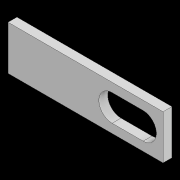
# Autodesk Inventor part: Platina Posterior Derecha
Saved by Autodesk Inventor 2021 (Build 250183000, 183)
## iProperties
Created: 2021-04-25
Part Number: Platina Posterior Derecha
Material: Generic
Document SubType Name: Modeling
Designer: maaro
Density: 1 g/cm^3
Appearance: Default
Author: maaro
Autodesk Inventor part; units mm, degrees
ref_plane "YZ Plane" through (0, 0, 0) normal (1, 0, 0) x (0, 1, 0)
ref_plane "XZ Plane" through (0, 0, 0) normal (0, 1, 0) x (-1, 0, 0)
ref_plane "XY Plane" through (0, 0, 0) normal (0, 0, 1) x (1, 0, 0)
sketch "Sketch1" plane through (0, 0, 0) normal (0, 0, 1) x (1, 0, 0)
  line L0 (-17.5, -5) -> (17.5, -5)
  line L1 (17.5, -5) -> (17.5, 5)
  line L2 (17.5, 5) -> (-17.5, 5)
  line L3 (-17.5, 5) -> (-17.5, -5)
  line L4 (-17.5, -5) -> (17.5, 5) construction
  line L5 (17.5, -5) -> (-17.5, 5) construction
  line L6 (6, 0) -> (13, 0) construction
  line L7 (6, -3) -> (13, -3)
  line L8 (13, 3) -> (6, 3)
  arc A0 (6, 3) -> (6, -3) centre (6, 0) ccw
  arc A1 (13, -3) -> (13, 3) centre (13, 0) ccw
  line L9 (-17.5, 0) -> (17.5, 0) construction
  point P0 (0, 0)
  point P1 (9.5, 0)
  dimension "d0" = 10
  dimension "d1" = 35
  dimension "d2" = 3
  dimension "d3" = 8
  dimension "d4" = 7
  constraints: 22 end point, 5 midpoint, 4 point on circle, 4 tangent, 3 parallel, 2 centre point, 2 horizontal, 1 collinear, 1 perpendicular
  measures "d0" distance of L0.end L1.end
  measures "d1" distance of L1.end L2.end
  measures "d2" distance from line of point (9.5, 0) L7
  measures "d3" distance from line of point (9.5, 0) L1
  measures "d4" distance of L6.end L6.start
extrude "Extrusion1" add sketch "Sketch1" along normal mid plane 2
body "Solid1"
